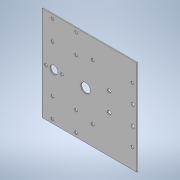
# Autodesk Inventor part: RD002_フレーム
Saved by Autodesk Inventor 2021 (Build 250183000, 183)
## iProperties
Created: 2020-10-26
Part Number: RD002_フレーム
Material: 一般
Document SubType Name: Modeling
Designer: ryusei
Density: 1 g/cm^3
Appearance: 既定
Author: ryusei
Autodesk Inventor part; units mm, degrees
ref_plane "YZ Plane" through (0, 0, 0) normal (1, 0, 0) x (0, 1, 0)
ref_plane "XZ Plane" through (0, 0, 0) normal (0, 1, 0) x (-1, 0, 0)
ref_plane "XY Plane" through (0, 0, 0) normal (0, 0, 1) x (1, 0, 0)
sketch "スケッチ1" plane through (0, 0, 0) normal (0, 0, 1) x (1, 0, 0)
  line L0 (0, 0) -> (120, 0)
  line L1 (120, 0) -> (120, 120)
  line L2 (120, 120) -> (0, 120)
  line L3 (0, 120) -> (0, 0)
  dimension "d1" = 120
  dimension "d2" = 120
  constraints: 8 end point, 2 parallel, 1 horizontal, 1 perpendicular
  measures "d1" distance between parallel lines of L0 L2
  measures "d2" distance between parallel lines of L1 L3
extrude "押し出し1" add sketch "スケッチ1" along normal blind 1
sketch "スケッチ2" plane through (0, 0, 1) normal (0, 0, 1) x (1, 0, 0)
  line L0 (0, 120) -> (0, 0) projected
  line L1 (0, 60) -> (120, 60) construction
  line L2 (120, 0) -> (120, 120) projected
  line L3 (120, 120) -> (0, 120) projected
  point P0 (13, 115)
  point P1 (13, 90)
  point P2 (43, 115)
  point P3 (43, 90)
  dimension "d8" = 13
  dimension "d9" = 5
  dimension "d12" = 25
  dimension "d15" = 30
  constraints: 2 end point, 2 midpoint, 1 horizontal, 1 vertical, 3 other
  measures "d8" distance from line of point (13, 115) L0
  measures "d9" distance from line of point (13, 115) L3
  measures "d12" distance of point (13, 115) point (13, 90)
  measures "d15" distance of point (13, 115) point (43, 115)
hole "穴1" at (13, 115, 1) at (13, 90, 1) at (43, 115, 1) at (43, 90, 1) direction (0, 0, -1) diameter 3.5 end through all
sketch "スケッチ3" plane through (0, 0, 1) normal (0, 0, 1) x (1, 0, 0)
  line L0 (0, 120) -> (0, 0) projected
  line L1 (0, 0) -> (120, 0) projected
  point P0 (13, 5)
  point P1 (43, 5)
  point P2 (13, 30)
  point P3 (43, 30)
  dimension "d25" = 13
  dimension "d26" = 5
  dimension "d29" = 30
  dimension "d32" = 25
  constraints: 1 horizontal, 1 vertical, 3 other
  measures "d25" distance from line of point (13, 5) L0
  measures "d26" distance from line of point (13, 5) L1
  measures "d29" distance of point (13, 5) point (43, 5)
  measures "d32" distance of point (13, 5) point (13, 30)
hole "穴2" at (13, 5, 1) at (43, 5, 1) at (13, 30, 1) at (43, 30, 1) direction (0, 0, -1) diameter 3.5 end through all
sketch "スケッチ4" plane through (0, 0, 1) normal (0, 0, 1) x (1, 0, 0)
  line L0 (0, 120) -> (0, 0) projected
  line L1 (0, 60) -> (120, 60) construction
  line L2 (120, 0) -> (120, 120) projected
  line L3 (120, 120) -> (0, 120) projected
  point P0 (5, 60)
  point P1 (25, 60)
  dimension "d42" = 5
  dimension "d43" = 60
  dimension "d46" = 20
  constraints: 2 end point, 2 midpoint, 1 horizontal, 1 point on line, 1 other
  measures "d42" distance of point (5, 60) L1.start
  measures "d43" distance from line of point (5, 60) L3
  measures "d46" distance of point (5, 60) point (25, 60)
hole "穴3" at (5, 60, 1) at (25, 60, 1) direction (0, 0, -1) diameter 3.5 end through all
sketch "スケッチ5" plane through (0, 0, 1) normal (0, 0, 1) x (1, 0, 0)
  line L0 (0, 120) -> (0, 0) projected
  line L1 (120, 120) -> (0, 120) projected
  point P0 (15, 60)
  dimension "d58" = 15
  dimension "d59" = 60
  measures "d58" distance from line of point (15, 60) L0
  measures "d59" distance from line of point (15, 60) L1
hole "穴4" at (15, 60, 1) direction (0, 0, -1) diameter 10 end through all
sketch "スケッチ6" plane through (0, 0, 1) normal (0, 0, 1) x (1, 0, 0)
  line L0 (0, 120) -> (0, 0) projected
  line L1 (120, 120) -> (0, 120) projected
  point P0 (55, 60)
  dimension "d67" = 55
  dimension "d68" = 60
  measures "d67" distance from line of L0 point (55, 60)
  measures "d68" distance from line of point (55, 60) L1
hole "穴5" at (55, 60, 1) direction (0, 0, -1) diameter 12 end through all
sketch "スケッチ7" plane through (0, 0, 1) normal (0, 0, 1) x (1, 0, 0)
  line L0 (0, 120) -> (0, 0) projected
  line L1 (0, 60) -> (120, 60) construction
  line L2 (120, 0) -> (120, 120) projected
  line L3 (120, 120) -> (0, 120) projected
  point P0 (64, 95.25)
  point P1 (64, 24.75)
  point P2 (114.2, 95.25)
  point P3 (114.2, 24.75)
  dimension "d76" = 64
  dimension "d77" = 24.75
  dimension "d80" = 70.5
  dimension "d83" = 50.2
  constraints: 2 end point, 2 midpoint, 1 horizontal, 1 vertical, 3 other
  measures "d76" distance from line of point (64, 95.25) L0
  measures "d77" distance from line of point (64, 95.25) L3
  measures "d80" distance of point (64, 95.25) point (64, 24.75)
  measures "d83" distance of point (64, 95.25) point (114.2, 95.25)
hole "穴6" at (64, 95.25, 1) at (64, 24.75, 1) at (114.2, 95.25, 1) at (114.2, 24.75, 1) direction (0, 0, -1) diameter 3.5 end through all
sketch "スケッチ8" plane through (0, 0, 1) normal (0, 0, 1) x (1, 0, 0)
  line L0 (0, 120) -> (0, 0) projected
  line L1 (120, 120) -> (0, 120) projected
  point P0 (85, 72)
  point P1 (85, 48)
  point P2 (115, 72)
  point P3 (115, 48)
  dimension "d93" = 85
  dimension "d94" = 48
  dimension "d97" = 24
  dimension "d100" = 30
  constraints: 1 horizontal, 1 vertical, 3 other
  measures "d93" distance from line of L0 point (85, 72)
  measures "d94" distance from line of point (85, 72) L1
  measures "d97" distance of point (85, 72) point (85, 48)
  measures "d100" distance of point (85, 72) point (115, 72)
hole "穴7" at (85, 72, 1) at (85, 48, 1) at (115, 72, 1) at (115, 48, 1) direction (0, 0, -1) diameter 4.5 end through all
